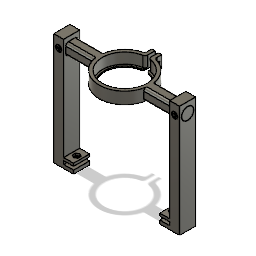
New DS Camera Capture Assembly v1 (Autodesk Fusion 360 design; units mm, degrees)
Autodesk Fusion 360 part; units mm, degrees
sketch "Sketch1" plane through (0, 0, 0) normal (0, 0, 1) x (1, 0, 0)
  line L0 (0, 0) -> (-15, 0)
  line L1 (-15, 0) -> (-15, 5.5)
  line L2 (-15, 5.5) -> (0, 5.5)
  line L3 (0, 5.5) -> (0, 0)
  line L4 (0, 0) -> (15, 0)
  line L5 (15, 0) -> (15, 180)
  line L6 (15, 180) -> (0, 180)
  line L7 (0, 180) -> (0, 0)
  line L8 (-15, 5.5) -> (0, 5.5)
  line L9 (0, 5.5) -> (0, 10.5)
  line L10 (0, 10.5) -> (-15, 10.5)
  line L11 (-15, 10.5) -> (-15, 5.5)
  line L12 (-15, 10.5) -> (0, 10.5)
  line L13 (0, 10.5) -> (0, 14.5)
  line L14 (0, 14.5) -> (-15, 14.5)
  line L15 (-15, 14.5) -> (-15, 10.5)
  dimension "d1" = 15
  dimension "d2" = 5.5
  dimension "d3" = 15
  dimension "d4" = 180
  dimension "d5" = 5
  dimension "d6" = 4
  constraint horizontal L0
  constraint vertical L1
  constraint horizontal L2
  constraint vertical L3
  constraint coincident L0.start L3.end
  constraint horizontal L4
  constraint vertical L5
  constraint horizontal L6
  constraint vertical L7
  constraint horizontal L8
  constraint vertical L9
  constraint horizontal L10
  constraint vertical L11
  constraint horizontal L12
  constraint vertical L13
  constraint horizontal L14
  constraint vertical L15
  measures "d1" distance of L0.start L0.end
  measures "d2" distance of L0.start L2.end
  measures "d3" distance of L0.start L4.end
  measures "d4" distance of L0.start L6.end
  measures "d5" distance of L1.end L10.end
  measures "d6" distance of L10.end L14.end
extrude "Extrude1" add sketch "Sketch1" along normal blind 24.5 contours L0 L1 L2 L3 L7 L8 | L3 L4 L5 L6 L7 L9 L13 | L7 L10 L12 L13 L14 L15 makes body 1
sketch "Sketch2" plane through (0, 14.5, 0) normal (0, 1, 0) x (-1, 0, 0)
  line L0 (0, 0) -> (15, 0)
  line L1 (15, 0) -> (15, 24.5)
  line L2 (15, 24.5) -> (0, 24.5)
  line L3 (0, 24.5) -> (0, 0)
  line L4 (7.5, 0) -> (7.5, 24.5)
  circle A0 centre (7.5, 12.25) radius 2.5
  dimension "d9" = 5
  constraint midpoint L0 L4.start
  constraint midpoint L2 L4.end
  constraint midpoint L4 A0.centre
  measures "d9" diameter of A0
extrude "Extrude2" cut sketch "Sketch2" against normal blind 14.5 contours L4 A0 | L4 A0 bodies 1
sketch "Sketch3" plane through (0, 14.5, 0) normal (0, 1, 0) x (-1, 0, 0)
  circle A0 centre (7.5, 12.25) radius 2.5
  line L0 (0, 0) -> (15, 0)
  line L1 (15, 0) -> (15, 24.5)
  line L2 (15, 24.5) -> (0, 24.5)
  line L3 (0, 24.5) -> (0, 0)
  line L4 (3.25, 9.7963) -> (7.5, 7.3425)
  line L5 (7.5, 7.3425) -> (11.75, 9.7963)
  line L6 (11.75, 9.7963) -> (11.75, 14.7037)
  line L7 (11.75, 14.7037) -> (7.5, 17.1575)
  line L8 (7.5, 17.1575) -> (3.25, 14.7037)
  line L9 (3.25, 14.7037) -> (3.25, 9.7963)
  point P0 (7.5, 12.25)
  dimension "d12" = 4.25
  constraint coincident P0 A0.centre
  measures "d12" distance of P0 L9
extrude "Extrude3" cut sketch "Sketch3" against normal blind 3.1 contours L4 L5 L6 L7 L8 L9 bodies 1
sketch "Sketch4" plane through (0, 0, 0) normal (-1, 0, 0) x (0, 0, 1)
  line L0 (0, 180) -> (0, 14.5)
  line L1 (0, 14.5) -> (24.5, 14.5)
  line L2 (24.5, 14.5) -> (24.5, 180)
  line L3 (24.5, 180) -> (0, 180)
  line L4 (12.25, 14.5) -> (12.25, 144.5)
  line L5 (12.25, 144.5) -> (17.25, 144.5)
  line L6 (21.25, 144.5) -> (7.25, 144.5)
  line L7 (3.25, 148.5) -> (3.25, 158.5)
  line L8 (7.25, 162.5) -> (17.25, 162.5)
  line L9 (21.25, 158.5) -> (21.25, 148.5)
  arc A0 (3.25, 148.5) -> (7.25, 144.5) centre (7.25, 148.5) ccw
  arc A1 (17.25, 144.5) -> (21.25, 148.5) centre (17.25, 148.5) ccw
  arc A2 (21.25, 158.5) -> (17.25, 162.5) centre (17.25, 158.5) ccw
  arc A3 (7.25, 162.5) -> (3.25, 158.5) centre (7.25, 158.5) ccw
  line L10 (24.5, 158.5) -> (0, 158.5)
  line L11 (0, 158.5) -> (0, 180)
  line L12 (0, 180) -> (24.5, 180)
  line L13 (24.5, 180) -> (24.5, 158.5)
  point P0 (3.25, 144.5)
  point P1 (21.25, 162.5)
  dimension "d15" = 130
  dimension "d16" = 9
  dimension "d17" = 18
  dimension "d18" = 18
  dimension "d19" = 4
  constraint midpoint L1 L4.start
  constraint perpendicular L1 L4
  constraint perpendicular L2 L5
  constraint horizontal L6
  constraint vertical L7
  constraint horizontal L8
  constraint vertical L9
  constraint coincident P0 L7
  constraint coincident P0 L6
  constraint tangent L7 A0
  constraint tangent L6 A0
  constraint coincident L6.start L5
  constraint coincident L6.start L9
  constraint tangent L5 A1
  constraint tangent L9 A1
  constraint equal A0 A1
  constraint coincident P1 L8
  constraint coincident P1 L9
  constraint tangent L8 A2
  constraint tangent L9 A2
  constraint equal A0 A2
  constraint tangent L7 A3
  constraint tangent L8 A3
  constraint equal A0 A3
  constraint horizontal L10
  constraint vertical L11
  constraint horizontal L12
  constraint vertical L13
  constraint coincident L0.start L3.end
  constraint coincident L2 L10.start
  measures "d15" distance of L4.start L4.end
  measures "d16" distance of L4.end L6.start
  measures "d17" distance of L6.start P0
  measures "d18" distance of L6.start P1
  measures "d19" radius of A0
extrude "Extrude4" cut sketch "Sketch4" against normal blind 15 contours L5 L6 L7 L9 A0 A1 L10 | L8 A2 A3 L10 bodies 1
sketch "Sketch5" plane through (0, 0, 0) normal (-1, 0, 0) x (0, 0, 1)
  line L0 (7.25, 162.5) -> (17.25, 162.5)
  arc A0 (21.25, 158.5) -> (17.25, 162.5) centre (17.25, 158.5) ccw
  line L1 (21.25, 158.5) -> (21.25, 148.5)
  arc A1 (17.25, 144.5) -> (21.25, 148.5) centre (17.25, 148.5) ccw
  line L2 (17.25, 144.5) -> (7.25, 144.5)
  arc A2 (3.25, 148.5) -> (7.25, 144.5) centre (7.25, 148.5) ccw
  line L3 (3.25, 148.5) -> (3.25, 158.5)
  arc A3 (7.25, 162.5) -> (3.25, 158.5) centre (7.25, 158.5) ccw
  line L4 (0, 180) -> (0, 14.5)
  line L5 (0, 14.5) -> (24.5, 14.5)
  line L6 (24.5, 14.5) -> (24.5, 180)
  line L7 (24.5, 180) -> (0, 180)
extrude "Extrude5" add sketch "Sketch5" along normal blind 160 separate body contours L0 A0 L1 A1 L2 A2 L3 A3 makes body 2
sketch "Sketch6" plane through (0, 0, 0) normal (-1, 0, 0) x (0, 0, 1)
  line L0 (7.25, 162.5) -> (17.25, 162.5)
  arc A0 (21.25, 158.5) -> (17.25, 162.5) centre (17.25, 158.5) ccw
  line L1 (21.25, 158.5) -> (21.25, 148.5)
  arc A1 (17.25, 144.5) -> (21.25, 148.5) centre (17.25, 148.5) ccw
  line L2 (17.25, 144.5) -> (7.25, 144.5)
  arc A2 (3.25, 148.5) -> (7.25, 144.5) centre (7.25, 148.5) ccw
  line L3 (3.25, 148.5) -> (3.25, 158.5)
  arc A3 (7.25, 162.5) -> (3.25, 158.5) centre (7.25, 158.5) ccw
  line L4 (0, 180) -> (0, 14.5)
  line L5 (0, 14.5) -> (24.5, 14.5)
  line L6 (24.5, 14.5) -> (24.5, 180)
  line L7 (24.5, 180) -> (0, 180)
  line L8 (21.25, 153.5) -> (3.25, 153.5)
  circle A4 centre (12.25, 153.5) radius 9
  constraint midpoint L1 L8.start
  constraint midpoint L3 L8.end
  constraint midpoint L8 A4.centre
  constraint tangent L2 A4
extrude "Extrude6" add sketch "Sketch6" against normal blind 15 contours L0 L3 A3 A4 | L0 A0 L1 A4 | L1 A1 L2 A4 | L2 A2 L3 A4 bodies 1
move_face "OffsetFaces1" offset -0.25 1 faces at (5, 154.3961, 21.2053) on bodies 1
sketch "Sketch7" plane through (0, 0, 0) normal (1, 0, 0) x (0, 0, -1)
  arc A0 (-17.25, 162.5) -> (-21.25, 158.5) centre (-17.25, 158.5) ccw
  line L0 (-21.25, 158.5) -> (-21.25, 148.5)
  arc A1 (-21.25, 148.5) -> (-17.25, 144.5) centre (-17.25, 148.5) ccw
  line L1 (-17.25, 144.5) -> (-7.25, 144.5)
  arc A2 (-7.25, 144.5) -> (-3.25, 148.5) centre (-7.25, 148.5) ccw
  line L2 (-3.25, 148.5) -> (-3.25, 158.5)
  arc A3 (-3.25, 158.5) -> (-7.25, 162.5) centre (-7.25, 158.5) ccw
  line L3 (-7.25, 162.5) -> (-17.25, 162.5)
  line L4 (-21.25, 153.5) -> (-3.25, 153.5)
  circle A4 centre (-12.25, 153.5) radius 9
  constraint midpoint L0 L4.start
  constraint midpoint L2 L4.end
  constraint midpoint L4 A4.centre
  constraint tangent L1 A4
extrude "Extrude7" add sketch "Sketch7" along normal blind 15 contours L4 A4 | L4 A4 bodies 2
extrude "Extrude8" cut 1 faces at (10, 180, 8.1667) along direction (0, -1, 0) blind 11 on bodies 1 bodies 1
sketch "Sketch8" plane through (0, 0, 0) normal (0, 0, -1) x (-1, 0, 0)
  line L0 (0, 169) -> (-15, 169)
  line L1 (-15, 169) -> (-15, 0)
  line L2 (-15, 0) -> (15, 0)
  line L3 (15, 0) -> (15, 5.5)
  line L4 (15, 5.5) -> (0, 5.5)
  line L5 (0, 5.5) -> (0, 10.5)
  line L6 (0, 10.5) -> (15, 10.5)
  line L7 (15, 10.5) -> (15, 14.5)
  line L8 (15, 14.5) -> (0, 14.5)
  line L9 (0, 14.5) -> (0, 169)
  line L10 (-7.5, 169) -> (-7.5, 162.75)
  line L11 (-7.5, 162.75) -> (-7.5, 144.25)
  circle A0 centre (-7.5, 153.5) radius 2.5
  dimension "d31" = 6.25
  dimension "d32" = 18.5
  dimension "d33" = 5
  constraint midpoint L0 L10.start
  constraint perpendicular L0 L10
  constraint parallel L10 L11
  constraint midpoint L11 A0.centre
  measures "d31" distance of L10.start L10.end
  measures "d32" distance of L10.end L11.end
  measures "d33" diameter of A0
extrude "Extrude9" cut sketch "Sketch8" against normal blind 24.5 contours L11 A0 | L11 A0 bodies 1 2
sketch "Sketch9" plane through (0, 0, 24.5) normal (0, 0, 1) x (1, 0, 0)
  circle A0 centre (7.5, 153.5) radius 2.5
  line L0 (15, 169) -> (0, 169)
  line L1 (0, 169) -> (0, 14.5)
  line L2 (0, 14.5) -> (-15, 14.5)
  line L3 (-15, 14.5) -> (-15, 10.5)
  line L4 (-15, 10.5) -> (0, 10.5)
  line L5 (0, 10.5) -> (0, 5.5)
  line L6 (0, 5.5) -> (-15, 5.5)
  line L7 (-15, 5.5) -> (-15, 0)
  line L8 (-15, 0) -> (15, 0)
  line L9 (15, 0) -> (15, 169)
  circle A1 centre (7.5, 153.5) radius 4.7
  dimension "d36" = 9.4
  constraint concentric A0 A1
  measures "d36" diameter of A1
extrude "Extrude10" cut sketch "Sketch9" against normal blind 2 contours A1 bodies 1
sketch "Sketch10" plane through (-160, 0, 0) normal (-1, 0, 0) x (0, 0, 1)
  arc A0 (21.25, 158.5) -> (17.25, 162.5) centre (17.25, 158.5) ccw
  line L0 (17.25, 162.5) -> (7.25, 162.5)
  arc A1 (7.25, 162.5) -> (3.25, 158.5) centre (7.25, 158.5) ccw
  line L1 (3.25, 158.5) -> (3.25, 148.5)
  arc A2 (3.25, 148.5) -> (7.25, 144.5) centre (7.25, 148.5) ccw
  line L2 (7.25, 144.5) -> (17.25, 144.5)
  arc A3 (17.25, 144.5) -> (21.25, 148.5) centre (17.25, 148.5) ccw
  line L3 (21.25, 148.5) -> (21.25, 158.5)
  line L4 (3.25, 153.5) -> (21.25, 153.5)
  circle A4 centre (12.25, 153.5) radius 9
  constraint midpoint L1 L4.start
  constraint midpoint L3 L4.end
  constraint midpoint L4 A4.centre
  constraint tangent L2 A4
extrude "Extrude11" add sketch "Sketch10" along normal blind 15 contours L4 A4 | L4 A4 bodies 2
sketch "Sketch11" plane through (0, 0, 3.25) normal (0, 0, -1) x (-1, 0, 0)
  line L0 (0, 153.5) -> (0, 148.5)
  line L1 (0, 148.5) -> (160, 148.5)
  line L2 (160, 148.5) -> (160, 153.5)
  line L3 (160, 153.5) -> (160, 158.5)
  line L4 (160, 158.5) -> (0, 158.5)
  line L5 (0, 158.5) -> (0, 153.5)
  line L6 (160, 158.5) -> (175, 158.5)
  line L7 (175, 158.5) -> (175, 148.5)
  line L8 (175, 148.5) -> (160, 148.5)
  line L9 (160, 148.5) -> (160, 158.5)
  line L10 (167.5, 158.5) -> (167.5, 148.5)
  circle A0 centre (167.5, 153.5) radius 2.5
  dimension "d41" = 15
  dimension "d42" = 10
  dimension "d43" = 5
  constraint horizontal L6
  constraint vertical L7
  constraint horizontal L8
  constraint vertical L9
  constraint coincident L3.end L4.start
  constraint midpoint L6 L10.start
  constraint midpoint L8 L10.end
  constraint midpoint L10 A0.centre
  measures "d41" distance of L3.end L6.end
  measures "d42" distance of L3.end L1.end
  measures "d43" diameter of A0
extrude "Extrude12" cut sketch "Sketch11" against normal blind 28 contours L10 A0 | L10 A0 bodies 2
sketch "Sketch12" plane through (0, 162.5, 0) normal (0, 1, 0) x (-1, 0, 0)
  line L0 (0, 12.25) -> (0, 7.25)
  line L1 (0, 7.25) -> (160, 7.25)
  line L2 (160, 7.25) -> (160, 12.25)
  line L3 (160, 12.25) -> (160, 17.25)
  line L4 (160, 17.25) -> (0, 17.25)
  line L5 (0, 17.25) -> (0, 12.25)
  line L6 (80, 7.25) -> (80, 17.25)
  circle A0 centre (80, 12.25) radius 33.75
  circle A1 centre (80, 12.25) radius 38.75
  dimension "d46" = 67.5
  dimension "d47" = 5
  constraint midpoint L1 L6.start
  constraint midpoint L4 L6.end
  constraint midpoint L6 A0.centre
  measures "d46" diameter of A0
extrude "Extrude13" cut sketch "Sketch12" against normal blind 50 contours L1 L4 L6 A0 | L1 A0 | L4 A0 | L1 L4 L6 A0 bodies 2 makes body 3 at (7.5, 150.1097, 20.587)
extrude "Extrude14" add sketch "Sketch12" against normal blind 18 contours L1 L4 A0 A1 | L1 A0 A1 | L4 A0 A1 | L1 L4 A0 A1 bodies 2 3
sketch "Sketch13" plane through (0, 162.5, 0) normal (0, 1, 0) x (-1, 0, 0)
  circle A0 centre (80, 12.25) radius 33.75
  arc A1 (118.4261, 17.25) -> (41.5739, 17.25) centre (80, 12.25) ccw
  line L0 (41.5739, 17.25) -> (0, 17.25)
  line L1 (0, 17.25) -> (0, 12.25)
  line L2 (0, 12.25) -> (0, 7.25)
  line L3 (0, 7.25) -> (41.5739, 7.25)
  arc A2 (41.5739, 7.25) -> (118.4261, 7.25) centre (80, 12.25) ccw
  line L4 (118.4261, 7.25) -> (160, 7.25)
  line L5 (160, 7.25) -> (160, 12.25)
  line L6 (160, 12.25) -> (160, 17.25)
  line L7 (160, 17.25) -> (118.4261, 17.25)
  line L8 (80, 12.25) -> (80, -26.5)
  line L9 (80, 12.25) -> (77.5, 12.25)
  line L10 (77.5, 12.25) -> (82.5, 12.25)
  line L11 (82.5, 12.25) -> (82.5, -36)
  line L12 (82.5, -36) -> (77.5, -36)
  line L13 (77.5, -36) -> (77.5, 12.25)
  dimension "d52" = 2.5
  dimension "d53" = 5
  constraint coincident A0.centre A1.centre
  constraint midpoint A2 L8.end
  constraint perpendicular L8 L9
  constraint horizontal L10
  constraint vertical L11
  constraint horizontal L12
  constraint vertical L13
  measures "d52" distance of A0.centre L9.end
  measures "d53" distance of L9.end L10.end
extrude "Extrude15" cut sketch "Sketch13" against normal blind 18 contours A0 L9 L10 L11 L13 | A0 A2 L8 L13 | A0 A2 L8 L11 bodies 2
sketch "Sketch14" plane through (0, 162.5, 0) normal (0, 1, 0) x (-1, 0, 0)
  line L0 (82.5, -21.4073) -> (82.5, -26.4193)
  arc A0 (82.5, -26.4193) -> (118.4261, 7.25) centre (80, 12.25) ccw
  line L1 (118.4261, 7.25) -> (160, 7.25)
  line L2 (160, 7.25) -> (160, 12.25)
  line L3 (160, 12.25) -> (160, 17.25)
  line L4 (160, 17.25) -> (118.4261, 17.25)
  arc A1 (118.4261, 17.25) -> (41.5739, 17.25) centre (80, 12.25) ccw
  line L5 (41.5739, 17.25) -> (0, 17.25)
  line L6 (0, 17.25) -> (0, 12.25)
  line L7 (0, 12.25) -> (0, 7.25)
  line L8 (0, 7.25) -> (41.5739, 7.25)
  arc A2 (41.5739, 7.25) -> (77.5, -26.4193) centre (80, 12.25) ccw
  line L9 (77.5, -26.4193) -> (77.5, -21.4073)
  arc A3 (82.5, -21.4073) -> (77.5, -21.4073) centre (80, 12.25) ccw
  line L10 (77.5, -21.4073) -> (72.5, -21.4073)
  line L11 (72.5, -21.4073) -> (72.5, -36.4073)
  line L12 (72.5, -36.4073) -> (77.5, -36.4073)
  line L13 (77.5, -36.4073) -> (77.5, -21.4073)
  line L14 (82.5, -21.4073) -> (87.5, -21.4073)
  line L15 (87.5, -21.4073) -> (87.5, -36.4073)
  line L16 (87.5, -36.4073) -> (82.5, -36.4073)
  line L17 (82.5, -36.4073) -> (82.5, -21.4073)
  dimension "d56" = 5
  dimension "d57" = 15
  dimension "d58" = 5
  dimension "d59" = 15
  constraint horizontal L10
  constraint vertical L11
  constraint horizontal L12
  constraint vertical L13
  constraint coincident L9.end A3.end
  constraint horizontal L14
  constraint vertical L15
  constraint horizontal L16
  constraint vertical L17
  constraint coincident L0.start A3.start
  measures "d56" distance of L9.end L10.end
  measures "d57" distance of L9.end L12.end
  measures "d58" distance of L0.start L14.end
  measures "d59" distance of L0.start L16.end
extrude "Extrude16" add sketch "Sketch14" against normal blind 18 contours A0 L15 L16 L17 | A2 L11 L12 L13 bodies 2
sketch "Sketch15" plane through (-72.5, 0, 0) normal (1, 0, 0) x (0, 0, -1)
  line L0 (36.4073, 162.5) -> (25.7673, 162.5)
  line L1 (25.7673, 162.5) -> (25.7673, 144.5)
  line L2 (25.7673, 144.5) -> (36.4073, 144.5)
  line L3 (36.4073, 144.5) -> (36.4073, 162.5)
  line L4 (25.7673, 153.5) -> (36.4073, 153.5)
  circle A0 centre (31.0873, 153.5) radius 2.5
  dimension "d62" = 5
  constraint midpoint L1 L4.start
  constraint midpoint L3 L4.end
  constraint midpoint L4 A0.centre
  measures "d62" diameter of A0
extrude "Extrude17" cut sketch "Sketch15" against normal blind 15 contours L4 A0 | L4 A0 bodies 2
sketch "Sketch16" plane through (-87.5, 0, 0) normal (-1, 0, 0) x (0, 0, 1)
  circle A0 centre (-31.0873, 153.5) radius 2.5
  line L0 (-25.7673, 162.5) -> (-36.4073, 162.5)
  line L1 (-36.4073, 162.5) -> (-36.4073, 144.5)
  line L2 (-36.4073, 144.5) -> (-25.7673, 144.5)
  line L3 (-25.7673, 144.5) -> (-25.7673, 162.5)
  line L4 (-26.5873, 156.0981) -> (-31.0873, 158.6962)
  line L5 (-31.0873, 158.6962) -> (-35.5873, 156.0981)
  line L6 (-35.5873, 156.0981) -> (-35.5873, 150.9019)
  line L7 (-35.5873, 150.9019) -> (-31.0873, 148.3038)
  line L8 (-31.0873, 148.3038) -> (-26.5873, 150.9019)
  line L9 (-26.5873, 150.9019) -> (-26.5873, 156.0981)
  point P0 (-31.0873, 153.5)
  dimension "d65" = 4.5
  constraint coincident P0 A0.centre
  measures "d65" distance of P0 L9
extrude "Extrude18" cut sketch "Sketch16" against normal blind 3.5 contours L4 L5 L6 L7 L8 L9 bodies 2
sketch "Sketch17" plane through (0, 144.5, 0) normal (0, -1, 0) x (1, 0, 0)
  line L0 (-77.5, -36.4073) -> (-72.5, -36.4073)
  line L1 (-72.5, -36.4073) -> (-72.5, -25.7673)
  arc A0 (-72.5, -25.7673) -> (-41.5739, 7.25) centre (-80, 12.25) ccw
  line L2 (-41.5739, 7.25) -> (0, 7.25)
  line L3 (0, 7.25) -> (0, 12.25)
  line L4 (0, 12.25) -> (0, 17.25)
  line L5 (0, 17.25) -> (-41.5739, 17.25)
  arc A1 (-41.5739, 17.25) -> (-118.4261, 17.25) centre (-80, 12.25) ccw
  line L6 (-118.4261, 17.25) -> (-160, 17.25)
  line L7 (-160, 17.25) -> (-160, 12.25)
  line L8 (-160, 12.25) -> (-160, 7.25)
  line L9 (-160, 7.25) -> (-118.4261, 7.25)
  arc A2 (-118.4261, 7.25) -> (-87.5, -25.7673) centre (-80, 12.25) ccw
  line L10 (-87.5, -25.7673) -> (-87.5, -36.4073)
  line L11 (-87.5, -36.4073) -> (-82.5, -36.4073)
  arc A3 (-77.5, -21.4073) -> (-82.5, -21.4073) centre (-80, 12.25) ccw
  arc A4 (-77.7222, -18.4155) -> (-82.2778, -18.4155) centre (-80, 12.25) ccw
  line L12 (-77.5, -21.4073) -> (-77.5, -18.3982)
  line L13 (-82.5, -21.4073) -> (-82.5, -18.3982)
  dimension "d68" = -3
  constraint coincident A3.start L12.start
  constraint coincident A4 L12.end
  constraint vertical L12
  constraint coincident A3.end L13.start
  constraint coincident A4 L13.end
  constraint parallel L12 L13
extrude "Extrude19" add sketch "Sketch17" against normal blind 2 bodies 2
fillet "Fillet1" radius 4 4 edges at (-77.5, 154.5, -21.4073) (-82.5, 154.5, -21.4073) (-87.5, 153.5, -25.7673) (-72.5, 153.5, -25.7673) on bodies 2
fillet "Fillet2" radius 4 2 edges at (-82.5, 145.5, -18.3982) (-77.5, 145.5, -18.3982) on bodies 2
mirror "Mirror1" about plane through (15, 0, 0) normal (1, 0, 0) of bodies 1 makes body 4
move_body "Move1" bodies 4 to x (1, 0, 0) y (0, 1, 0) z (0, 0, 1) at (-190, 0, 0)
equation "d12 = ( 8.5 / 2 ) * 1 mm"
equation "d29 = -16 mm + 5 mm"
equation "d65 = ( 9 / 2 ) * 1 mm"
